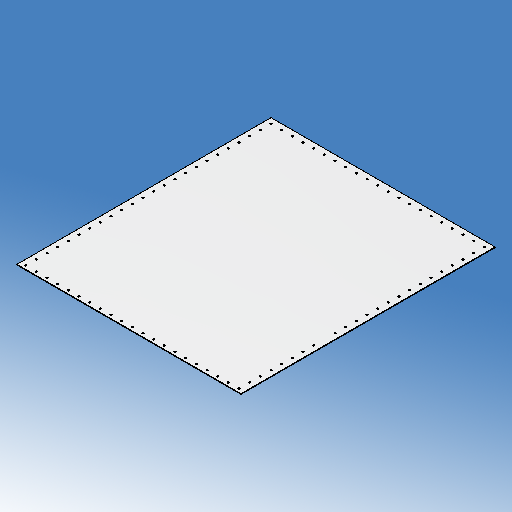
# Autodesk Inventor part: EBox-BottomPlate
Saved by Autodesk Inventor 2025 (Build 290162000, 162)
## iProperties
Created: 2023-01-19
Part Number: EBox-BottomPlate
Material: Aluminum 6061
Document SubType Name: Modeling
Designer: Nebil
Density: 2.7 g/cm^3
Appearance: Aluminum - Flat
Author: Nebil
Autodesk Inventor part; units mm, degrees
ref_plane "YZ Plane" through (0, 0, 0) normal (1, 0, 0) x (0, 1, 0)
ref_plane "XZ Plane" through (0, 0, 0) normal (0, 1, 0) x (-1, 0, 0)
ref_plane "XY Plane" through (0, 0, 0) normal (0, 0, 1) x (1, 0, 0)
sketch "Sketch1" plane through (0, 0, 0) normal (0, 1, 0) x (-1, 0, 0)
  line L0 (-266.7, 302.514) -> (266.7, 302.514)
  line L1 (266.7, 302.514) -> (266.7, -302.514)
  line L2 (266.7, -302.514) -> (-266.7, -302.514)
  line L3 (-266.7, -302.514) -> (-266.7, 302.514)
  line L4 (-266.7, 302.514) -> (266.7, -302.514) construction
  line L5 (266.7, 302.514) -> (-266.7, -302.514) construction
  circle A0 centre (254, -289.814) radius 2.0701
  circle A1 centre (228.6, -289.814) radius 2.0701
  circle A2 centre (203.2, -289.814) radius 2.0701
  circle A3 centre (177.8, -289.814) radius 2.0701
  circle A4 centre (152.4, -289.814) radius 2.0701
  circle A5 centre (127, -289.814) radius 2.0701
  circle A6 centre (101.6, -289.814) radius 2.0701
  circle A7 centre (76.2, -289.814) radius 2.0701
  circle A8 centre (50.8, -289.814) radius 2.0701
  circle A9 centre (254, -264.414) radius 2.0701
  circle A10 centre (254, -239.014) radius 2.0701
  circle A11 centre (254, -213.614) radius 2.0701
  circle A12 centre (254, -188.214) radius 2.0701
  circle A13 centre (254, -162.814) radius 2.0701
  circle A14 centre (254, -137.414) radius 2.0701
  circle A15 centre (254, -112.014) radius 2.0701
  circle A16 centre (254, -86.614) radius 2.0701
  circle A17 centre (254, -61.214) radius 2.0701
  circle A18 centre (254, -35.814) radius 2.0701
  circle A19 centre (254, -10.414) radius 2.0701
  circle A20 centre (254, 14.986) radius 2.0701
  circle A21 centre (254, 40.386) radius 2.0701
  circle A22 centre (254, 65.786) radius 2.0701
  circle A23 centre (254, 91.186) radius 2.0701
  circle A24 centre (254, 116.586) radius 2.0701
  circle A25 centre (254, 141.986) radius 2.0701
  circle A26 centre (254, 167.386) radius 2.0701
  circle A27 centre (254, 192.786) radius 2.0701
  circle A28 centre (254, 218.186) radius 2.0701
  circle A29 centre (254, 243.586) radius 2.0701
  circle A30 centre (254, 268.986) radius 2.0701
  circle A31 centre (254, 294.386) radius 2.0701
  circle A32 centre (228.6, 294.386) radius 2.0701
  circle A33 centre (203.2, 294.386) radius 2.0701
  circle A34 centre (177.8, 294.386) radius 2.0701
  circle A35 centre (152.4, 294.386) radius 2.0701
  circle A36 centre (127, 294.386) radius 2.0701
  circle A37 centre (101.6, 294.386) radius 2.0701
  circle A38 centre (76.2, 294.386) radius 2.0701
  circle A39 centre (50.8, 294.386) radius 2.0701
  circle A40 centre (154.4701, -175.514) radius 38.1 construction
  circle A41 centre (25.4, -289.814) radius 2.0701
  circle A42 centre (0, -289.814) radius 2.0701
  circle A43 centre (-25.4, -289.814) radius 2.0701
  circle A44 centre (-50.8, -289.814) radius 2.0701
  circle A45 centre (-76.2, -289.814) radius 2.0701
  circle A46 centre (-101.6, -289.814) radius 2.0701
  circle A47 centre (-127, -289.814) radius 2.0701
  circle A48 centre (-152.4, -289.814) radius 2.0701
  circle A49 centre (-177.8, -289.814) radius 2.0701
  circle A50 centre (-203.2, -289.814) radius 2.0701
  circle A51 centre (-228.6, -289.814) radius 2.0701
  circle A52 centre (25.4, 294.386) radius 2.0701
  circle A53 centre (0, 294.386) radius 2.0701
  circle A54 centre (-25.4, 294.386) radius 2.0701
  circle A55 centre (-50.8, 294.386) radius 2.0701
  circle A56 centre (-76.2, 294.386) radius 2.0701
  circle A57 centre (-101.6, 294.386) radius 2.0701
  circle A58 centre (-127, 294.386) radius 2.0701
  circle A59 centre (-152.4, 294.386) radius 2.0701
  circle A60 centre (-177.8, 294.386) radius 2.0701
  circle A61 centre (-203.2, 294.386) radius 2.0701
  circle A62 centre (-228.6, 294.386) radius 2.0701
  line L6 (0, -302.514) -> (0, 302.514) construction
  circle A63 centre (-254, -289.814) radius 2.0701
  circle A64 centre (-254, -264.414) radius 2.0701
  circle A65 centre (-254, -239.014) radius 2.0701
  circle A66 centre (-254, -213.614) radius 2.0701
  circle A67 centre (-254, -188.214) radius 2.0701
  circle A68 centre (-254, -162.814) radius 2.0701
  circle A69 centre (-254, -137.414) radius 2.0701
  circle A70 centre (-254, -112.014) radius 2.0701
  circle A71 centre (-254, -86.614) radius 2.0701
  circle A72 centre (-254, -61.214) radius 2.0701
  circle A73 centre (-254, -35.814) radius 2.0701
  circle A74 centre (-254, -10.414) radius 2.0701
  circle A75 centre (-254, 14.986) radius 2.0701
  circle A76 centre (-254, 40.386) radius 2.0701
  circle A77 centre (-254, 65.786) radius 2.0701
  circle A78 centre (-254, 116.586) radius 2.0701
  circle A79 centre (-254, 141.986) radius 2.0701
  circle A80 centre (-254, 167.386) radius 2.0701
  circle A81 centre (-254, 192.786) radius 2.0701
  circle A82 centre (-254, 218.186) radius 2.0701
  circle A83 centre (-254, 243.586) radius 2.0701
  circle A84 centre (-254, 268.986) radius 2.0701
  circle A85 centre (-254, 294.386) radius 2.0701
  point P0 (0, 0)
  dimension "d0" = 605.028
  dimension "d1" = 533.4
  dimension "d5" = 4.1402
  dimension "d6" = 12.7
  dimension "d7" = 12.7
  dimension "d10" = 25.4
  dimension "d17" = 25.4
  dimension "d24" = 25.4
  dimension "d36" = 76.2
  dimension "d37" = 127
  constraints: 86 centre point, 23 symmetric about line, 14 end point, 4 midpoint, 3 horizontal, 2 parallel, 1 perpendicular, 1 vertical, 145 other
  measures "d0" distance of L0.end L1.end
  measures "d1" distance of L1.end L2.end
  measures "d5" diameter of A0
  measures "d6" distance from line of A0.centre L2
  measures "d7" distance from line of L1 A0.centre
  measures "d10" distance of A0.centre A1.centre
  measures "d17" distance of A0.centre A9.centre
  measures "d24" distance of A31.centre A32.centre
  measures "d36" diameter of A40
  measures "d37" distance from line of A40.centre L2
extrude "Extrusion1" add sketch "Sketch1" along normal blind 1.5875
body "Solid1"
